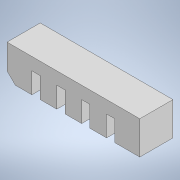
# Autodesk Inventor part: body
Saved by Autodesk Inventor 2021 (Build 250183000, 183)
## iProperties
Created: 2022-01-02
Part Number: body
Material: 一般
Document SubType Name: Modeling
Designer: shibu
Density: 1 g/cm^3
Appearance: 既定
Author: shibu
Autodesk Inventor part; units mm, degrees
ref_plane "YZ Plane" through (0, 0, 0) normal (1, 0, 0) x (0, 1, 0)
ref_plane "XZ Plane" through (0, 0, 0) normal (0, 1, 0) x (-1, 0, 0)
ref_plane "XY Plane" through (0, 0, 0) normal (0, 0, 1) x (1, 0, 0)
sketch "スケッチ1" plane through (0, 0, 0) normal (0, 0, 1) x (1, 0, 0)
  line L0 (0, 0) -> (-15, 0)
  line L1 (-15, 0) -> (-15, 20)
  line L2 (-15, 20) -> (0, 20)
  line L3 (0, 20) -> (0, 0)
  line L4 (0, 0) -> (0, 43.6966) construction
  line L5 (-15, 12.5) -> (-20, 12.5)
  line L6 (-20, 12.5) -> (-20, 0)
  line L7 (-30, 0) -> (-30, 12.5)
  line L8 (-30, 0) -> (-20, 0)
  line L9 (23.8812, 0) -> (-169.724, 0) construction
  line L10 (-45, 0) -> (-45, 12.5)
  line L11 (-45, 0) -> (-35, 0)
  line L12 (-35, 12.5) -> (-35, 0)
  line L13 (-30, 12.5) -> (-35, 12.5)
  line L14 (-60, 0) -> (-60, 12.5)
  line L15 (-60, 0) -> (-50, 0)
  line L16 (-50, 12.5) -> (-50, 0)
  line L17 (-45, 12.5) -> (-50, 12.5)
  line L18 (-75, 0) -> (-75, 12.5)
  line L19 (-75, 0) -> (-65, 0)
  line L20 (-65, 12.5) -> (-65, 0)
  line L21 (-60, 12.5) -> (-65, 12.5)
  line L22 (-75, 0) -> (-80, 0)
  line L23 (-80, 0) -> (-80, 20)
  line L24 (-80, 20) -> (-75, 20)
  line L25 (-75, 20) -> (-75, 0)
  line L26 (-75, 20) -> (-15, 20)
  line L27 (-75, 0) -> (-80, 5)
  line L28 (-75, 0) -> (-67.9289, 0) construction
  line L29 (0, 5) -> (-5, 0)
  point P0 (-5, 0)
  dimension "d1" = 15
  dimension "d2" = 20
  dimension "d3" = 5
  dimension "d4" = 10
  dimension "d5" = 7.5
  dimension "d8" = 15
  dimension "d13" = 5
  dimension "d14" = 135
  dimension "d15" = 5
  dimension "d16" = 135
  constraints: 60 end point, 9 point on line, 5 collinear, 5 horizontal, 4 parallel, 4 perpendicular, 1 equal length, 1 vertical, 27 other
  measures "d1" distance of L1.end L2.end
  measures "d2" distance of L0.end L1.end
  measures "d3" distance of L5.start L5.end
  measures "d4" distance between parallel lines of L6 L7
  measures "d5" distance between parallel lines of L5 L2
  measures "d8" distance of L7.start L10.start
  measures "d13" distance of L23.end L24.end
  measures "d14" angle of L28 L27
  measures "d15" distance from line of L9 L29.start
  measures "d16" angle of L0 L29
extrude "押し出し1" add sketch "スケッチ1" along normal blind 10 contours L0 L29 L3 | L0 L1 L2 L3 L29 | L5 L6 L8 L7 L13 L12 L11 L10 L17 L16 L15 L14 L21 L20 L19 L18 L25 L26 L1 | L25 L18 L27 L23 L24
sketch "スケッチ2" plane through (0, 0, 0) normal (0, 0, -1) x (-1, 0, 0)
  line L0 (80, 20) -> (80, 5) projected
  line L1 (0, 20) -> (80, 20) projected
  line L2 (0, 0) -> (0, 20) projected
  line L3 (15, 0) -> (0, 0) projected
  line L4 (15, 12.5) -> (15, 0) projected
  line L5 (20, 12.5) -> (15, 12.5) projected
  line L6 (20, 0) -> (20, 12.5) projected
  line L7 (30, 0) -> (20, 0) projected
  line L8 (30, 12.5) -> (30, 0) projected
  line L9 (35, 12.5) -> (30, 12.5) projected
  line L10 (35, 0) -> (35, 12.5) projected
  line L11 (45, 0) -> (35, 0) projected
  line L12 (45, 12.5) -> (45, 0) projected
  line L13 (50, 12.5) -> (45, 12.5) projected
  line L14 (50, 0) -> (50, 12.5) projected
  line L15 (60, 0) -> (50, 0) projected
  line L16 (60, 12.5) -> (60, 0) projected
  line L17 (65, 12.5) -> (60, 12.5) projected
  line L18 (65, 0) -> (65, 12.5) projected
  line L19 (75, 0) -> (65, 0) projected
  line L20 (80, 5) -> (75, 0) projected
  line L21 (40, 31.6917) -> (40, -9.5966) construction
  line L22 (42.5, 5) -> (37.5, 5)
  line L23 (37.5, 5) -> (37.5, 17.5)
  line L24 (37.5, 17.5) -> (42.5, 17.5)
  line L25 (42.5, 17.5) -> (42.5, 5)
  line L26 (42.5, 5) -> (37.5, 17.5) construction
  line L27 (37.5, 5) -> (42.5, 17.5) construction
  line L28 (-3.4293, 0) -> (98.1355, 0) construction
  line L29 (52.5, 5) -> (52.5, 17.5)
  line L30 (57.5, 5) -> (52.5, 5)
  line L31 (57.5, 17.5) -> (57.5, 5)
  line L32 (67.5, 5) -> (67.5, 17.5)
  line L33 (72.5, 5) -> (67.5, 5)
  line L34 (72.5, 17.5) -> (72.5, 5)
  line L35 (22.5, 5) -> (22.5, 17.5)
  line L36 (27.5, 5) -> (22.5, 5)
  line L37 (27.5, 17.5) -> (27.5, 5)
  line L38 (37.5, 5) -> (37.5, 17.5)
  line L39 (42.5, 5) -> (37.5, 5)
  line L40 (42.5, 17.5) -> (42.5, 5)
  line L41 (52.5, 5) -> (52.5, 17.5)
  line L42 (57.5, 5) -> (52.5, 5)
  line L43 (57.5, 17.5) -> (57.5, 5)
  line L44 (7.5, 5) -> (7.5, 17.5)
  line L45 (12.5, 5) -> (7.5, 5)
  line L46 (12.5, 17.5) -> (12.5, 5)
  line L47 (22.5, 5) -> (22.5, 17.5)
  line L48 (27.5, 5) -> (22.5, 5)
  line L49 (27.5, 17.5) -> (27.5, 5)
  line L50 (37.5, 5) -> (37.5, 17.5)
  line L51 (42.5, 5) -> (37.5, 5)
  line L52 (42.5, 17.5) -> (42.5, 5)
  line L53 (72.5, 17.5) -> (7.5, 17.5)
  line L54 (7.5, 15) -> (72.5, 15)
  point P0 (40, 11.25)
  point P1 (12.5, 15)
  point P2 (22.5, 15)
  point P3 (27.5, 15)
  point P4 (37.5, 15)
  point P5 (42.5, 15)
  point P6 (52.5, 15)
  point P7 (57.5, 15)
  point P8 (67.5, 15)
  dimension "d19" = 5
  dimension "d20" = 5
  dimension "d21" = 12.5
  dimension "d22" = 5
  dimension "d25" = 15
  dimension "d28" = 15
  dimension "d31" = 2.5
  constraints: 68 end point, 6 horizontal, 4 point on line, 2 midpoint, 2 parallel, 1 perpendicular, 1 vertical, 56 other
  measures "d19" distance between parallel lines of L12 L21
  measures "d20" distance of L23.end L24.end
  measures "d21" distance of L22.end L23.end
  measures "d22" distance between parallel lines of L11 L22
  measures "d25" distance of L22.end L29.start
  measures "d28" distance of L22.end L35.start
  measures "d31" distance between parallel lines of L54 L53
extrude "押し出し2" cut sketch "スケッチ2" against normal blind 7.5 contours L22 L23 L54 L25 | L54 L23 L24 L25 | L25 L53 L29 L54 | L54 L37 L53 L23 | L54 L31 L30 L29 | L29 L53 L31 L54 | L54 L35 L53 L37 | L37 L36 L35 L54 | L31 L53 L32 L54 | L54 L46 L53 L35 | L54 L34 L33 L32 | L32 L53 L34 L54 | L54 L44 L53 L46 | L46 L45 L44 L54
mirror "ミラー2" about plane through (-40, 10, 0) normal (0, 0, -1) of "押し出し1", "押し出し2"
